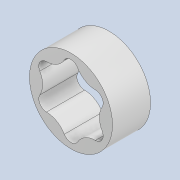
# Autodesk Inventor part: 原動節接続部v2外
Saved by Autodesk Inventor 2020.4 (Build 244396000, 396)
## iProperties
Created: 2021-02-21
Part Number: 原動節接続部v2外
Material: アルミニウム 2014-T4
Document SubType Name: Modeling
Designer: AA19065
Density: 2.8 g/cm^3
Appearance: サテン
Mass: 0.71358 g
Surface Area: 4.79717 cm^2
Volume: 0.25485 cm^3
Author: AA19065
Autodesk Inventor part; units mm, degrees
ref_plane "YZ Plane" through (0, 0, 0) normal (1, 0, 0) x (0, 1, 0)
ref_plane "XZ Plane" through (0, 0, 0) normal (0, 1, 0) x (-1, 0, 0)
ref_plane "XY Plane" through (0, 0, 0) normal (0, 0, 1) x (1, 0, 0)
sketch "スケッチ1" plane through (0, 0, 0) normal (0, 0, 1) x (1, 0, 0)
  circle A0 centre (-12.7279, -12.7279) radius 6
  arc A1 (-11.767, -8.0827) -> (-12.7279, -7.5279) centre (-12.7279, -8.6375) ccw
  arc A2 (-12.7279, -7.5279) -> (-13.6889, -8.0827) centre (-12.7279, -8.6375) ccw
  arc A3 (-16.2703, -9.5731) -> (-13.6889, -8.0827) centre (-16.2703, -6.5923) ccw
  arc A4 (-16.2703, -9.5731) -> (-17.2313, -10.1279) centre (-16.2703, -10.6827) ccw
  arc A5 (-17.2313, -10.1279) -> (-17.2313, -11.2375) centre (-16.2703, -10.6827) ccw
  arc A6 (-17.2313, -14.2183) -> (-17.2313, -11.2375) centre (-19.8127, -12.7279) ccw
  arc A7 (-17.2313, -14.2183) -> (-17.2313, -15.3279) centre (-16.2703, -14.7731) ccw
  arc A8 (-17.2313, -15.3279) -> (-16.2703, -15.8827) centre (-16.2703, -14.7731) ccw
  arc A9 (-13.6889, -17.3731) -> (-16.2703, -15.8827) centre (-16.2703, -18.8635) ccw
  arc A10 (-13.6889, -17.3731) -> (-12.7279, -17.9279) centre (-12.7279, -16.8183) ccw
  arc A11 (-12.7279, -17.9279) -> (-11.767, -17.3731) centre (-12.7279, -16.8183) ccw
  arc A12 (-9.1855, -15.8827) -> (-11.767, -17.3731) centre (-9.1855, -18.8635) ccw
  arc A13 (-9.1855, -15.8827) -> (-8.2246, -15.3279) centre (-9.1855, -14.7731) ccw
  arc A14 (-8.2246, -15.3279) -> (-8.2246, -14.2183) centre (-9.1855, -14.7731) ccw
  arc A15 (-8.2246, -11.2375) -> (-8.2246, -14.2183) centre (-5.6431, -12.7279) ccw
  arc A16 (-8.2246, -11.2375) -> (-8.2246, -10.1279) centre (-9.1855, -10.6827) ccw
  arc A17 (-8.2246, -10.1279) -> (-9.1855, -9.5731) centre (-9.1855, -10.6827) ccw
  arc A18 (-11.767, -8.0827) -> (-9.1855, -9.5731) centre (-9.1855, -6.5923) ccw
  point P0 (0, 0)
  point P1 (0, 0)
  constraints: 36 point on circle, 19 centre point, 66 other
extrude "押し出し1" add sketch "スケッチ1" along normal blind 5.5
sketch "書き出し" plane through (-12.7279, -12.7279, 5.5) normal (0, 0, 1) x (1, 0, 0)
  circle A0 centre (0, 0) radius 6 projected
  arc A1 (4.5033, 1.4904) -> (4.5033, -1.4904) centre (7.0848, 0) ccw projected
  arc A2 (3.5424, -3.1548) -> (4.5033, -1.4904) centre (3.5424, -2.0452) ccw projected
  arc A3 (3.5424, -3.1548) -> (0.9609, -4.6452) centre (3.5424, -6.1356) ccw projected
  arc A4 (-0.9609, -4.6452) -> (0.9609, -4.6452) centre (0, -4.0904) ccw projected
  arc A5 (-0.9609, -4.6452) -> (-3.5424, -3.1548) centre (-3.5424, -6.1356) ccw projected
  arc A6 (-4.5033, -1.4904) -> (-3.5424, -3.1548) centre (-3.5424, -2.0452) ccw projected
  arc A7 (-4.5033, -1.4904) -> (-4.5033, 1.4904) centre (-7.0848, 0) ccw projected
  arc A8 (-3.5424, 3.1548) -> (-4.5033, 1.4904) centre (-3.5424, 2.0452) ccw projected
  arc A9 (-3.5424, 3.1548) -> (-0.9609, 4.6452) centre (-3.5424, 6.1356) ccw projected
  arc A10 (0.9609, 4.6452) -> (-0.9609, 4.6452) centre (0, 4.0904) ccw projected
  arc A11 (0.9609, 4.6452) -> (3.5424, 3.1548) centre (3.5424, 6.1356) ccw projected
  arc A12 (4.5033, 1.4904) -> (3.5424, 3.1548) centre (3.5424, 2.0452) ccw projected
  point P0 (12.7279, 12.7279)
